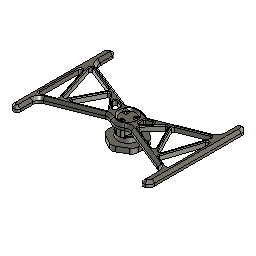
SL1S Form Wash Adapter v1 (Autodesk Fusion 360 design; units mm, degrees)
Autodesk Fusion 360 part; units mm, degrees
sketch "Sketch1" plane through (0, 0, 0) normal (0, 0, 1) x (1, 0, 0)
  line L0 (0, 21.131) -> (-18.3, 10.5655)
  line L1 (-18.3, 10.5655) -> (-18.3, -10.5655)
  line L2 (-18.3, -10.5655) -> (0, -21.131)
  line L3 (0, -21.131) -> (18.3, -10.5655)
  line L4 (18.3, -10.5655) -> (18.3, 10.5655)
  line L5 (18.3, 10.5655) -> (0, 21.131)
  dimension "d1" = 36.6
  constraint vertical L1
  measures "d1" distance of L1 L4
extrude "Extrude1" add sketch "Sketch1" along normal blind 6 makes body 1
fillet "Fillet1" radius 8 6 edges at (-18.3, -10.5655, 3) (-18.3, 10.5655, 3) (0, 21.131, 3) (18.3, 10.5655, 3) (0, -21.131, 3) (18.3, -10.5655, 3) on bodies 1
sketch "Sketch2" plane through (0, 0, 6) normal (0, 0, 1) x (-1, 0, 0)
  line L0 (-18.3, 5.9467) -> (-18.3, -5.9467)
  line L1 (-14.3, -12.8749) -> (-4, -18.8216)
  line L2 (4, -18.8216) -> (14.3, -12.8749)
  line L3 (18.3, -5.9467) -> (18.3, 5.9467)
  line L4 (14.3, 12.8749) -> (4, 18.8216)
  line L5 (-4, 18.8216) -> (-14.3, 12.8749)
  circle A0 centre (0, 0) radius 12
  arc A1 (-14.3, 12.8749) -> (-18.3, 5.9467) centre (-10.3, 5.9467) ccw
  arc A2 (-18.3, -5.9467) -> (-14.3, -12.8749) centre (-10.3, -5.9467) ccw
  arc A3 (-4, -18.8216) -> (4, -18.8216) centre (0, -11.8934) ccw
  arc A4 (14.3, -12.8749) -> (18.3, -5.9467) centre (10.3, -5.9467) ccw
  arc A5 (18.3, 5.9467) -> (14.3, 12.8749) centre (10.3, 5.9467) ccw
  arc A6 (4, 18.8216) -> (-4, 18.8216) centre (0, 11.8934) ccw
  dimension "d6" = 24
  constraint coincident A0.centre origin
  measures "d6" diameter of A0
extrude "Extrude2" add sketch "Sketch2" along normal blind 5 contours A0 bodies 1
sketch "Sketch3" plane through (0, 0, 11) normal (0, 0, 1) x (-1, 0, 0)
  circle A0 centre (0, 0) radius 12
  line L0 (0, -60) -> (-84, -60)
  line L1 (-84, -60) -> (-84, 60)
  line L2 (-84, 60) -> (0, 60)
  line L3 (0, 60) -> (0, -60)
  line L4 (-74, -60) -> (-74, 60)
  circle A1 centre (0, 0) radius 15
  line L5 (-11.1803, -10) -> (-74, -35)
  line L6 (-11.1803, 10) -> (-74, 35)
  line L7 (-13.878, -5.6922) -> (-74, -29.6186)
  line L8 (-13.878, 5.6922) -> (-74, 29.6186)
  line L9 (-74, 29.6186) -> (-78, 31.2105)
  line L10 (-78, 31.2105) -> (-78, -31.2105)
  line L11 (-78, -31.2105) -> (-74, -29.6186)
  line L12 (-13.878, -5.6922) -> (-13.878, 5.6922)
  line L13 (-78, -31.2105) -> (-60.0405, 24.0632)
  line L14 (-57.2473, 22.9516) -> (-74.3772, -29.7687)
  line L15 (-57.2473, 22.9516) -> (-37.8015, -15.2129)
  line L16 (-53.0239, 21.2709) -> (-35.0022, -14.0988)
  line L17 (-35.0022, -14.0988) -> (-16.8299, 6.8669)
  line L18 (-13.878, 5.6922) -> (-28.9415, -11.6869)
  line L19 (-35.0022, -14.0988) -> (-35.0022, 14.0988) construction
  dimension "d9" = 84
  dimension "d10" = 60
  dimension "d11" = 60
  dimension "d12" = 10
  dimension "d13" = 30
  dimension "d14" = 10
  dimension "d15" = 10
  dimension "d16" = 25
  dimension "d17" = 25
  dimension "d18" = 5
  dimension "d19" = 5
  dimension "d20" = 4
  dimension "d21" = 3
  dimension "d22" = 3
  dimension "d23" = 3
  dimension "d24" = 18
  dimension "d25" = 45
  constraint horizontal L0
  constraint vertical L1
  constraint horizontal L2
  constraint vertical L3
  constraint coincident A0.centre L3
  constraint coincident L0 L4.start
  constraint coincident L2 L4.end
  constraint perpendicular L2 L4
  constraint coincident A0.centre A1.centre
  constraint coincident A1 L5.start
  constraint coincident L4 L5.end
  constraint coincident L4 L6.end
  constraint coincident A1 L6.start
  constraint coincident A1 L7.start
  constraint coincident L4 L7.end
  constraint parallel L5 L7
  constraint coincident A1 L8.start
  constraint coincident L4 L8.end
  constraint parallel L6 L8
  constraint parallel L8 L9
  constraint parallel L1 L10
  constraint parallel L7 L11
  constraint coincident L8 L13.end
  constraint coincident L8 L14.start
  constraint coincident L7 L14.end
  constraint parallel L13 L14
  constraint coincident L7 L15.end
  constraint coincident L8 L16.start
  constraint coincident L7 L16.end
  constraint parallel L15 L16
  constraint coincident L8 L17.end
  constraint parallel L17 L18
  constraint coincident L7 L18.end
  constraint coincident L8 L19.end
  constraint vertical L19
  measures "d9" distance of L0.start L0.end
  measures "d10" distance of A0.centre L0
  measures "d11" distance of A0.centre L2
  measures "d12" distance of L1 L4
  measures "d13" diameter of A1
  measures "d14" vertical distance of A0.centre L6.start
  measures "d15" vertical distance of A0.centre L5.start
  measures "d16" distance of L4.start L5.end
  measures "d17" distance of L4.end L6.end
  measures "d18" distance of L5 L7
  measures "d19" distance of L6 L8
  measures "d20" distance of L4 L10
  measures "d21" distance of L17 L18
  measures "d22" distance of L15 L16
  measures "d23" distance of L13 L14
  measures "d24" angle of L10 L13
  measures "d25" angle of L14 L15
extrude "Extrude3" add sketch "Sketch3" along normal blind 6 separate body contours A0 L3 | A0 L3 A1 L12 | L4 A1 L6 L8 | L4 A1 L5 L7 | L0 L1 L2 L4 L9 L10 L11 | L7 L8 L17 L18 | L7 L8 L15 L16 | L4 L8 L13 L14 | L4 L11 L13 L14 picked at (-5.459, -1.0652) makes body 2
fillet "Fillet2" radius 2 12 edges at (78, 31.2105, 14) (78, -31.2105, 14) (74.3772, 29.7687, 14) (57.2473, -22.9516, 14) (37.8015, 15.2129, 14) (35.0022, 14.0988, 14) (28.9415, 11.6869, 14) (13.878, 5.6922, 14) (13.878, -5.6922, 14) (16.8299, -6.8669, 14) (53.0239, -21.2709, 14) (60.0405, -24.0632, 14) on bodies 2
fillet "Fillet3" radius 8 4 edges at (11.1803, -10, 14) (11.1803, 10, 14) (74, 35, 14) (74, -35, 14) on bodies 2
fillet "Fillet4" radius 8 2 edges at (84, -60, 14) (84, 60, 14) on bodies 2
chamfer "Chamfer1" distance 3 angle 45 10 edges at (42.2896, -22.3804, 17) (72.6206, -35.9357, 17) (74, -50.2133, 17) (4.3111, -14.3671, 17) (11.8472, -11.242, 17) (42.2896, 22.3804, 17) (11.8472, 11.242, 17) (4.3111, 14.3671, 17) (74, 50.2133, 17) (72.6206, 35.9357, 17) on bodies 2
chamfer "Chamfer2" distance 1 angle 45 24 edges at (68.5215, -27.4383, 17) (60.7116, -23.7482, 17) (67.3589, -1.5396, 17) (76.3129, 20.5583, 17) (78, -4.8395, 17) (77.1227, -29.9171, 17) (56.9942, -19.7353, 17) (65.9001, 3.6789, 17) (72.5265, 27.7944, 17) (55.1296, 22.1089, 17) (38.7081, 14.8712, 17) (46.9264, -2.6958, 17) (50.3107, -18.7976, 17) (43.4825, -2.5448, 17) (34.8107, 12.5301, 17) (25.8654, 3.5576, 17) (18.2418, -6.523, 17) (33.7693, -13.6082, 17) (15.1789, -2.205, 17) (20.4768, 1.9209, 17) (23.6833, 7.9513, 17) (18.2259, 7.4225, 17) (14.2229, 5.4583, 17) (13.878, 2.0022, 17) on bodies 2
fillet "Fillet5" radius 4 2 edges at (74, -60, 12.5) (74, 60, 12.5) on bodies 2
chamfer "Chamfer3" distance 3 angle 45 5 edges at (84, 0, 17) (82.9282, 56, 17) (78.5402, 59.4275, 17) (78.5402, -59.4275, 17) (82.9282, -56, 17) on bodies 2
move_body "Move1" bodies 1 to x (1, 0, 0) y (0, 1, 0) z (0, 0, 1) at (0, 0, -10)
sketch "Sketch4" plane through (0, 0, 1) normal (0, 0, 1) x (-1, 0, 0)
  circle A0 centre (0, 0) radius 12
extrude "Extrude4" add sketch "Sketch4" along normal blind 10 separate body makes body 3
sketch "Sketch5" plane through (0, 0, 11) normal (0, 0, 1) x (-1, 0, 0)
  circle A0 centre (0, 0) radius 12
  circle A1 centre (0, -20) radius 12.5
  line L0 (0, -20) -> (0, 0)
  dimension "d41" = 25
  dimension "d42" = 20
  constraint coincident A1.centre L0.start
  constraint coincident A0.centre L0.end
  constraint vertical L0
  measures "d41" diameter of A1
  measures "d42" distance of A1.centre A0.centre
extrude "Extrude5" cut sketch "Sketch5" against normal blind 10 contours A0 A1 L0 | A0 A1 L0 bodies 3
pattern_circular "C-Pattern1" count 3 over 360 about axis through (0, 0, 11) along (0, 0, 1) of "Extrude5"
mirror "Mirror1" about plane through (0, -12, 11) normal (-1, 0, 0) of bodies 2 merged
sketch "Sketch6" plane through (0, 0, 17) normal (0, 0, 1) x (-1, 0, 0)
  arc A0 (51.5056, 16.0883) -> (47.7233, 20.2377) centre (48.8326, 17.4503) ccw
  line L0 (51.5056, 16.0883) -> (37.2414, -11.9068)
  arc A1 (32.3014, -12.5097) -> (37.2414, -11.9068) centre (34.5684, -10.5448) ccw
  line L1 (32.3014, -12.5097) -> (17.918, 4.0847)
  arc A2 (19.0757, 8.837) -> (17.918, 4.0847) centre (20.185, 6.0496) ccw
  line L2 (19.0757, 8.837) -> (47.7233, 20.2377)
  line L3 (61.4127, 25.6856) -> (74.8907, 31.0494)
  arc A3 (79, 28.262) -> (74.8907, 31.0494) centre (76, 28.262) ccw
  line L4 (79, 28.262) -> (79, -18.583)
  arc A4 (73.1468, -19.51) -> (79, -18.583) centre (76, -18.583) ccw
  line L5 (73.1468, -19.51) -> (59.6688, 21.9711)
  arc A5 (61.4127, 25.6856) -> (59.6688, 21.9711) centre (62.522, 22.8982) ccw
  arc A6 (59.6904, 18.6685) -> (54.1642, 19.1034) centre (56.8372, 17.7415) ccw
  line L6 (59.6904, 18.6685) -> (74.0118, -25.4082)
  arc A7 (70.0494, -29.1227) -> (74.0118, -25.4082) centre (71.1586, -26.3353) ccw
  line L7 (70.0494, -29.1227) -> (39.4703, -16.9533)
  arc A8 (37.9066, -12.8039) -> (39.4703, -16.9533) centre (40.5796, -14.1659) ccw
  line L8 (37.9066, -12.8039) -> (54.1642, 19.1034)
  arc A9 (18.145, 2.2961) -> (12.878, 0.3312) centre (15.878, 0.3312) ccw
  line L9 (18.145, 2.2961) -> (24.3199, -4.828)
  arc A10 (20.9436, -9.5803) -> (24.3199, -4.828) centre (22.0529, -6.7929) ccw
  line L10 (20.9436, -9.5803) -> (14.7687, -7.1229)
  arc A11 (12.878, -4.3356) -> (14.7687, -7.1229) centre (15.878, -4.3356) ccw
  line L11 (12.878, -4.3356) -> (12.878, 0.3312)
  arc A12 (-12.878, 0.3312) -> (-18.145, 2.2961) centre (-15.878, 0.3312) ccw
  line L12 (-12.878, 0.3312) -> (-12.878, -4.3356)
  arc A13 (-14.7687, -7.1229) -> (-12.878, -4.3356) centre (-15.878, -4.3356) ccw
  line L13 (-14.7687, -7.1229) -> (-20.9436, -9.5803)
  arc A14 (-24.3199, -4.828) -> (-20.9436, -9.5803) centre (-22.0529, -6.7929) ccw
  line L14 (-24.3199, -4.828) -> (-18.145, 2.2961)
  arc A15 (-54.1642, 19.1034) -> (-59.6904, 18.6685) centre (-56.8372, 17.7415) ccw
  line L15 (-54.1642, 19.1034) -> (-37.9066, -12.8039)
  arc A16 (-39.4703, -16.9533) -> (-37.9066, -12.8039) centre (-40.5796, -14.1659) ccw
  line L16 (-39.4703, -16.9533) -> (-70.0494, -29.1227)
  arc A17 (-74.0118, -25.4082) -> (-70.0494, -29.1227) centre (-71.1586, -26.3353) ccw
  line L17 (-74.0118, -25.4082) -> (-59.6904, 18.6685)
  arc A18 (-77, 55.4641) -> (-78.5, 56.3301) centre (-78, 55.4641) ccw
  arc A19 (-78.5, 56.3301) -> (-81, 52) centre (-76, 52) ccw
  line L18 (-81, 52) -> (-81, -52)
  arc A20 (-81, -52) -> (-78.5, -56.3301) centre (-76, -52) ccw
  arc A21 (-78.5, -56.3301) -> (-77, -55.4641) centre (-78, -55.4641) ccw
  line L19 (-77, -55.4641) -> (-77, -40.4265)
  arc A22 (-70.0674, -30.2061) -> (-77, -40.4265) centre (-66, -40.4265) ccw
  line L20 (-70.0674, -30.2061) -> (-16.7303, -8.9799)
  arc A23 (-6.6068, -10.0175) -> (-16.7303, -8.9799) centre (-12.6629, -19.2003) ccw
  arc A24 (-6.6068, -10.0175) -> (6.6068, -10.0175) centre (0, 0) ccw
  arc A25 (16.7303, -8.9799) -> (6.6068, -10.0175) centre (12.6629, -19.2003) ccw
  line L21 (16.7303, -8.9799) -> (70.0674, -30.2061)
  arc A26 (77, -40.4265) -> (70.0674, -30.2061) centre (66, -40.4265) ccw
  line L22 (77, -40.4265) -> (77, -55.4641)
  arc A27 (77, -55.4641) -> (78.5, -56.3301) centre (78, -55.4641) ccw
  arc A28 (78.5, -56.3301) -> (81, -52) centre (76, -52) ccw
  line L23 (81, -52) -> (81, 52)
  arc A29 (81, 52) -> (78.5, 56.3301) centre (76, 52) ccw
  arc A30 (78.5, 56.3301) -> (77, 55.4641) centre (78, 55.4641) ccw
  line L24 (77, 55.4641) -> (77, 40.4265)
  arc A31 (70.0674, 30.2061) -> (77, 40.4265) centre (66, 40.4265) ccw
  line L25 (70.0674, 30.2061) -> (16.7303, 8.9799)
  arc A32 (6.6068, 10.0175) -> (16.7303, 8.9799) centre (12.6629, 19.2003) ccw
  arc A33 (6.6068, 10.0175) -> (-6.6068, 10.0175) centre (0, 0) ccw
  arc A34 (-16.7303, 8.9799) -> (-6.6068, 10.0175) centre (-12.6629, 19.2003) ccw
  line L26 (-16.7303, 8.9799) -> (-70.0674, 30.2061)
  arc A35 (-77, 40.4265) -> (-70.0674, 30.2061) centre (-66, 40.4265) ccw
  line L27 (-77, 40.4265) -> (-77, 55.4641)
  line L28 (-74.8907, 31.0494) -> (-61.4127, 25.6856)
  arc A36 (-59.6688, 21.9711) -> (-61.4127, 25.6856) centre (-62.522, 22.8982) ccw
  line L29 (-59.6688, 21.9711) -> (-73.1468, -19.51)
  arc A37 (-79, -18.583) -> (-73.1468, -19.51) centre (-76, -18.583) ccw
  line L30 (-79, -18.583) -> (-79, 28.262)
  arc A38 (-74.8907, 31.0494) -> (-79, 28.262) centre (-76, 28.262) ccw
  arc A39 (-47.7233, 20.2377) -> (-51.5056, 16.0883) centre (-48.8326, 17.4503) ccw
  line L31 (-47.7233, 20.2377) -> (-19.0757, 8.837)
  arc A40 (-17.918, 4.0847) -> (-19.0757, 8.837) centre (-20.185, 6.0496) ccw
  line L32 (-17.918, 4.0847) -> (-32.3014, -12.5097)
  arc A41 (-37.2414, -11.9068) -> (-32.3014, -12.5097) centre (-34.5684, -10.5448) ccw
  line L33 (-37.2414, -11.9068) -> (-51.5056, 16.0883)
  circle A42 centre (0, 0) radius 11
  dimension "d49" = 22
  constraint concentric A24 A42
  measures "d49" diameter of A42
extrude "Extrude6" cut sketch "Sketch6" against normal blind 2 contours A42 bodies 2
chamfer "Chamfer4" distance 2 angle 45 1 edges at (10.2556, -3.9778, 15) on bodies 2
sketch "Sketch7" plane through (0, 0, 15) normal (0, 0, 1) x (-1, 0, 0)
  circle A0 centre (0, 0) radius 9
  circle A1 centre (0, 0) radius 7.5 construction
  circle A2 centre (0, 7.5) radius 3
  line L0 (0, 7.5) -> (0, 0) construction
  dimension "d53" = 15
  dimension "d54" = 6
  constraint concentric A0 A1
  constraint coincident A1 A2.centre
  constraint coincident A2.centre L0.start
  constraint coincident A0.centre A1.centre
  constraint vertical L0
  measures "d53" diameter of A1
  measures "d54" diameter of A2
extrude "Extrude7" cut sketch "Sketch7" along normal blind 40 and the other way blind 1 contours A0 A2 | A0 A2 picked at (-0.033, 7.4884) picked at (0.0713, 9.4854) bodies 2
pattern_circular "C-Pattern2" count 3 over 360 about axis through (0, 0, 15) along (0, 0, -1) of "Extrude7"
hole "Hole1" at (0, -7.5, 14) direction (0, 0, -1) diameter 3.2 depth 52 tip angle 118 bodies 1 2 3
pattern_circular "C-Pattern3" count 3 over 360 about axis through (0, 0, 15) along (0, 0, -1) of "Hole1"
hole "Hole2" at (0, -7.5, -10) direction (0, 0, 1) diameter 3.2 depth 52 tip angle 118 counterbore diameter 5 counterbore depth 6 bodies 1
sketch "Sketch8" plane through (0, 0, 11) normal (0, 0, -1) x (1, 0, 0)
  circle A0 centre (6.4952, -3.75) radius 1.6
  circle A1 centre (-6.4952, -3.75) radius 1.6
  circle A2 centre (0, 7.5) radius 1.6
  arc A3 (-13.878, 0.3312) -> (-17.3893, 1.6411) centre (-15.878, 0.3312) ccw
  line L0 (-13.878, 0.3312) -> (-13.878, -4.3356)
  arc A4 (-15.1385, -6.1938) -> (-13.878, -4.3356) centre (-15.878, -4.3356) ccw
  line L1 (-15.1385, -6.1938) -> (-21.3134, -8.6512)
  arc A5 (-23.5642, -5.483) -> (-21.3134, -8.6512) centre (-22.0529, -6.7929) ccw
  line L2 (-23.5642, -5.483) -> (-17.3893, 1.6411)
  arc A6 (-18.6737, 4.7396) -> (-19.4455, 7.9078) centre (-20.185, 6.0496) ccw
  line L3 (-18.6737, 4.7396) -> (-33.0571, -11.8548)
  arc A7 (-36.3504, -11.4528) -> (-33.0571, -11.8548) centre (-34.5684, -10.5448) ccw
  line L4 (-36.3504, -11.4528) -> (-50.6146, 16.5423)
  arc A8 (-48.0931, 19.3086) -> (-50.6146, 16.5423) centre (-48.8326, 17.4503) ccw
  line L5 (-48.0931, 19.3086) -> (-19.4455, 7.9078)
  arc A9 (-39.8401, -16.0242) -> (-38.7976, -13.2579) centre (-40.5796, -14.1659) ccw
  line L6 (-39.8401, -16.0242) -> (-70.4191, -28.1935)
  arc A10 (-73.0608, -25.7173) -> (-70.4191, -28.1935) centre (-71.1586, -26.3353) ccw
  line L7 (-73.0608, -25.7173) -> (-58.7394, 18.3595)
  arc A11 (-55.0552, 18.6495) -> (-58.7394, 18.3595) centre (-56.8372, 17.7415) ccw
  line L8 (-55.0552, 18.6495) -> (-38.7976, -13.2579)
  arc A12 (-60.6198, 22.2802) -> (-61.7824, 24.7564) centre (-62.522, 22.8982) ccw
  line L9 (-60.6198, 22.2802) -> (-74.0979, -19.201)
  arc A13 (-78, -18.583) -> (-74.0979, -19.201) centre (-76, -18.583) ccw
  line L10 (-78, -18.583) -> (-78, 28.262)
  arc A14 (-75.2605, 30.1202) -> (-78, 28.262) centre (-76, 28.262) ccw
  line L11 (-75.2605, 30.1202) -> (-61.7824, 24.7564)
  arc A15 (61.7824, 24.7564) -> (60.6198, 22.2802) centre (62.522, 22.8982) ccw
  line L12 (61.7824, 24.7564) -> (75.2605, 30.1202)
  arc A16 (78, 28.262) -> (75.2605, 30.1202) centre (76, 28.262) ccw
  line L13 (78, 28.262) -> (78, -18.583)
  arc A17 (74.0979, -19.201) -> (78, -18.583) centre (76, -18.583) ccw
  line L14 (74.0979, -19.201) -> (60.6198, 22.2802)
  arc A18 (38.7976, -13.2579) -> (39.8401, -16.0242) centre (40.5796, -14.1659) ccw
  line L15 (38.7976, -13.2579) -> (55.0552, 18.6495)
  arc A19 (58.7394, 18.3595) -> (55.0552, 18.6495) centre (56.8372, 17.7415) ccw
  line L16 (58.7394, 18.3595) -> (73.0608, -25.7173)
  arc A20 (70.4191, -28.1935) -> (73.0608, -25.7173) centre (71.1586, -26.3353) ccw
  line L17 (70.4191, -28.1935) -> (39.8401, -16.0242)
  arc A21 (19.4455, 7.9078) -> (18.6737, 4.7396) centre (20.185, 6.0496) ccw
  line L18 (19.4455, 7.9078) -> (48.0931, 19.3086)
  arc A22 (50.6146, 16.5423) -> (48.0931, 19.3086) centre (48.8326, 17.4503) ccw
  line L19 (50.6146, 16.5423) -> (36.3504, -11.4528)
  arc A23 (33.0571, -11.8548) -> (36.3504, -11.4528) centre (34.5684, -10.5448) ccw
  line L20 (33.0571, -11.8548) -> (18.6737, 4.7396)
  arc A24 (17.3893, 1.6411) -> (13.878, 0.3312) centre (15.878, 0.3312) ccw
  line L21 (17.3893, 1.6411) -> (23.5642, -5.483)
  arc A25 (21.3134, -8.6512) -> (23.5642, -5.483) centre (22.0529, -6.7929) ccw
  line L22 (21.3134, -8.6512) -> (15.1385, -6.1938)
  arc A26 (13.878, -4.3356) -> (15.1385, -6.1938) centre (15.878, -4.3356) ccw
  line L23 (13.878, -4.3356) -> (13.878, 0.3312)
  arc A27 (74, -55.4641) -> (80, -58.9282) centre (78, -55.4641) ccw
  arc A28 (80, -58.9282) -> (84, -52) centre (76, -52) ccw
  line L24 (84, -52) -> (84, 52)
  arc A29 (84, 52) -> (80, 58.9282) centre (76, 52) ccw
  arc A30 (80, 58.9282) -> (74, 55.4641) centre (78, 55.4641) ccw
  line L25 (74, 55.4641) -> (74, 40.4265)
  arc A31 (68.9581, 32.9935) -> (74, 40.4265) centre (66, 40.4265) ccw
  line L26 (68.9581, 32.9935) -> (15.621, 11.7672)
  arc A32 (8.2584, 12.5219) -> (15.621, 11.7672) centre (12.6629, 19.2003) ccw
  arc A33 (8.2584, 12.5219) -> (-8.2584, 12.5219) centre (0, 0) ccw
  arc A34 (-15.621, 11.7672) -> (-8.2584, 12.5219) centre (-12.6629, 19.2003) ccw
  line L27 (-15.621, 11.7672) -> (-68.9581, 32.9935)
  arc A35 (-74, 40.4265) -> (-68.9581, 32.9935) centre (-66, 40.4265) ccw
  line L28 (-74, 40.4265) -> (-74, 55.4641)
  arc A36 (-74, 55.4641) -> (-80, 58.9282) centre (-78, 55.4641) ccw
  arc A37 (-80, 58.9282) -> (-84, 52) centre (-76, 52) ccw
  line L29 (-84, 52) -> (-84, -52)
  arc A38 (-84, -52) -> (-80, -58.9282) centre (-76, -52) ccw
  arc A39 (-80, -58.9282) -> (-74, -55.4641) centre (-78, -55.4641) ccw
  line L30 (-74, -55.4641) -> (-74, -40.4265)
  arc A40 (-68.9581, -32.9935) -> (-74, -40.4265) centre (-66, -40.4265) ccw
  line L31 (-68.9581, -32.9935) -> (-15.621, -11.7672)
  arc A41 (-8.2584, -12.5219) -> (-15.621, -11.7672) centre (-12.6629, -19.2003) ccw
  arc A42 (-8.2584, -12.5219) -> (8.2584, -12.5219) centre (0, 0) ccw
  arc A43 (15.621, -11.7672) -> (8.2584, -12.5219) centre (12.6629, -19.2003) ccw
  line L32 (15.621, -11.7672) -> (68.9581, -32.9935)
  arc A44 (74, -40.4265) -> (68.9581, -32.9935) centre (66, -40.4265) ccw
  line L33 (74, -40.4265) -> (74, -55.4641)
  circle A45 centre (6.4952, -3.75) radius 1.6
  circle A46 centre (-6.4952, -3.75) radius 1.6
  circle A47 centre (0, 7.5) radius 1.6
  arc A48 (11.9317, -1.2788) -> (4.8584, 10.9725) centre (17.3205, 10) cw
  arc A49 (4.8584, 10.9725) -> (-4.8584, 10.9725) centre (0, 0) ccw
  arc A50 (-4.8584, 10.9725) -> (-11.9317, -1.2788) centre (-17.3205, 10) cw
  arc A51 (-11.9317, -1.2788) -> (-7.0733, -9.6938) centre (0, 0) ccw
  arc A52 (-7.0733, -9.6937) -> (7.0733, -9.6937) centre (0, -20) cw
  arc A53 (7.0733, -9.6938) -> (11.9317, -1.2788) centre (0, 0) ccw
  circle A54 centre (0, 0) radius 12.5
  line L34 (4.8584, 10.9725) -> (4.8995, 11.4998)
  line L35 (11.9317, -1.2788) -> (12.4089, -1.5068)
  dimension "d71" = 25
  constraint concentric A33 A54
  constraint coincident A48.end A49.start
  constraint coincident A54 L34.end
  constraint tangent A48 L34
  constraint coincident A48.start A53.end
  constraint coincident A54 L35.end
  constraint tangent A48 L35
  measures "d71" diameter of A54
extrude "Extrude8" cut sketch "Sketch8" against normal blind 2 contours A48 A54 L34 L35 bodies 2
fillet "Fillet6" radius 0.5 2 edges at (4.8995, -11.4998, 12) (12.4089, 1.5068, 12) on bodies 2
chamfer "Chamfer5" distance 0.5 angle 45 4 edges at (6.4952, -3.75, 13) (5.0936, -11.1776, 13) (10.8253, -6.25, 13) (12.2269, 1.1776, 13) on bodies 2
pattern_circular "C-Pattern4" count 3 over 360 about axis through (0, 0, 17) along (0, 0, -1) of "Extrude8", "Fillet6", "Chamfer5"
sketch "Sketch9" plane through (0, 0, 1) normal (0, 0, 1) x (-1, 0, 0)
  circle A0 centre (-6.4952, -3.75) radius 1.6
  circle A1 centre (6.4952, -3.75) radius 1.6
  circle A2 centre (0, 7.5) radius 1.6
  circle A3 centre (0, 0) radius 12
  arc A4 (-11.9317, -1.2788) -> (-4.8584, 10.9725) centre (-17.3205, 10) ccw
  arc A5 (-12.0394, -1.0532) -> (-5.1076, 10.9531) centre (-17.3205, 10) ccw
  dimension "d79" = -0.25
extrude "Extrude9" add sketch "Sketch9" along normal blind 1.5 contours A3 A5 bodies 1
fillet "Fillet7" radius 1 2 edges at (5.1009, -10.8619, 1.75) (11.9571, 1.0135, 1.75) on bodies 1
chamfer "Chamfer6" distance 0.5 angle 45 4 edges at (10.3923, -6, 2.5) (11.4724, 0.1598, 2.5) (6.7117, -3.875, 2.5) (5.5978, -10.0153, 2.5) on bodies 1
pattern_circular "C-Pattern5" count 3 over 360 about axis through (0, 0, 1) along (0, 0, 1) of "Extrude9", "Fillet7", "Chamfer6"
fillet "Fillet8" radius 3 6 edges at (4.8584, -10.9725, 6) (-4.8584, -10.9725, 6) (11.9317, 1.2788, 6) (7.0733, 9.6938, 6) (-7.0733, 9.6938, 6) (-11.9317, 1.2788, 6) on bodies 3
pattern_circular "C-Pattern6" count 3 over 360 about axis through (0, 0, -4) along (0, 0, -1) of "Hole2"
equation "d19 = d18"
equation "d22 = d21"
equation "d23 = d21"
named bodies: "SFWA_Insert", "SFWA_Bracket", "SFWA_Spacer"
